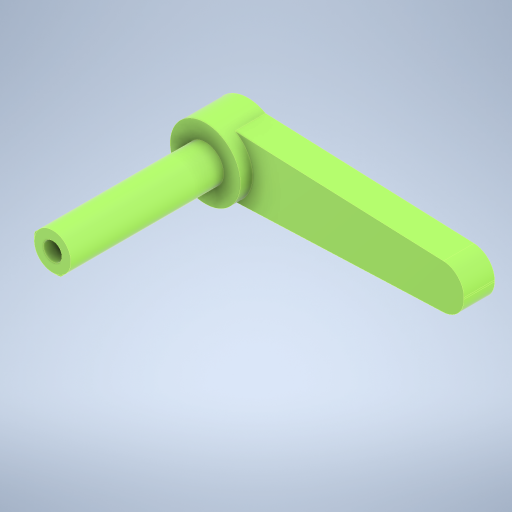
# Autodesk Inventor part: Right leg distributor
Saved by Autodesk Inventor 2023 (Build 270158000, 158)
## iProperties
Created: 2022-05-02
Part Number: Right leg distributor
Material: Phenolic Resin
Document SubType Name: Modeling
Designer: Devin
Density: 1.38 g/cm^3
Appearance: Light Green
Author: Devin
Autodesk Inventor part; units mm, degrees
ref_plane "YZ Plane" through (0, 0, 0) normal (1, 0, 0) x (0, 1, 0)
ref_plane "XZ Plane" through (0, 0, 0) normal (0, 1, 0) x (-1, 0, 0)
ref_plane "XY Plane" through (0, 0, 0) normal (0, 0, 1) x (1, 0, 0)
sketch "Sketch1" plane through (0, 0, 0) normal (0, 0, 1) x (1, 0, 0)
  arc A0 (1.4424, 2.54) -> (1.4424, -2.54) centre (0, 0) ccw
  line L0 (1.4424, 2.54) -> (18.7855, 1.8463)
  line L1 (18.7855, -1.8463) -> (1.4424, -2.54)
  line L2 (20.4924, 0.0697) -> (20.4924, -0.0697)
  arc A1 (18.7855, -1.8463) -> (20.4924, -0.0697) centre (18.7144, -0.0697) ccw
  arc A2 (20.4924, 0.0697) -> (18.7855, 1.8463) centre (18.7144, 0.0697) ccw
  point P0 (20.4924, 1.778)
  point P1 (20.4924, -1.778)
  point P2 (20.4924, 0)
  dimension "d0" = 5.842
  dimension "d1" = 5.08
  dimension "d2" = 3.556
  dimension "d3" = 1.778
  dimension "d4" = 19.05
  dimension "d5" = 1.778
  constraints: 6 end point, 6 point on circle, 4 tangent, 3 centre point, 3 point on line, 3 vertical alignment, 1 coincident, 1 equal radius, 1 horizontal alignment, 1 vertical
  measures "d0" diameter of A0
  measures "d1" distance of L1.end L0.start
  measures "d2" distance of point (20.492, -1.778) point (20.492, 1.778)
  measures "d3" distance of point (20.492, -1.778) point (20.492, 0)
  measures "d4" horizontal distance of point (20.492, 1.778) L0.start
  measures "d5" radius of A1
extrude "Extrusion1" add sketch "Sketch1" along normal blind 2.54
sketch "Sketch2" plane through (0, 0, 2.54) normal (0, 0, 1) x (1, 0, 0)
  circle A0 centre (0, 0) radius 2.921
  constraints: 1 centre point, 1 coincident
extrude "Extrusion2" add sketch "Sketch2" along normal blind 1.016
sketch "Sketch3" plane through (0, 0, 3.556) normal (0, 0, 1) x (1, 0, 0)
  circle A0 centre (0, 0) radius 0.762
  circle A1 centre (0, 0) radius 1.524
  dimension "d10" = 1.524
  dimension "d11" = 0.762
  constraints: 2 centre point, 1 coincident
  measures "d10" diameter of A0
  measures "d11" radial gap between concentric circles of A0 A1
extrude "Extrusion3" add sketch "Sketch3" along normal blind 12.7
sketch "Sketch4" plane through (0, 0, 3.556) normal (0, 0, 1) x (1, 0, 0)
  circle A0 centre (0, 0) radius 1.524 projected
  line L0 (-1.0776, 1.0776) -> (-1.7252, 0.4301)
  line L1 (1.0776, -1.0776) -> (0.4301, -1.7252)
  arc A1 (-1.7252, 0.4301) -> (0.4301, -1.7252) centre (0, 0) ccw
  arc A2 (-1.0776, 1.0776) -> (1.0776, -1.0776) centre (0, 0) ccw
  dimension "d17" = 3.302
  constraints: 4 end point, 4 point on circle, 2 centre point, 2 tangent
extrude "Extrusion5" add sketch "Sketch4" along normal blind 12.446 contours A0 L1 A1 L0
body "Solid1"
